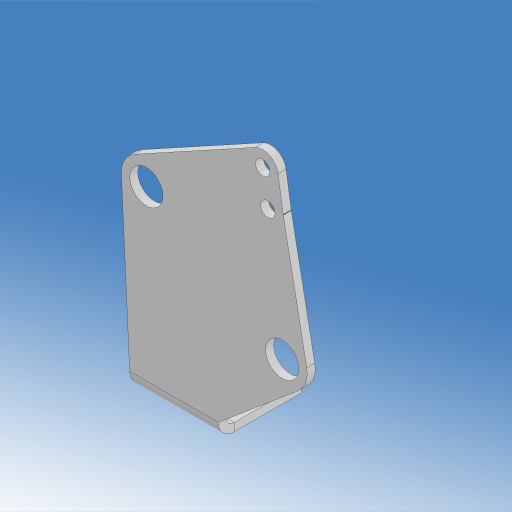
# Autodesk Inventor part: GearsMount
Saved by Autodesk Inventor 2024 (Build 280153000, 153)
## iProperties
Created: 2024-03-12
Part Number: GearsMount
Material: Generic
Document SubType Name: Sheet Metal
Designer: seene
Density: 1 g/cm^3
Sheet Metal Rule: Default
Appearance: Default
Author: seene
Autodesk Inventor part; units mm, degrees
ref_plane "YZ Plane" through (0, 0, 0) normal (1, 0, 0) x (0, 1, 0)
ref_plane "XZ Plane" through (0, 0, 0) normal (0, 1, 0) x (-1, 0, 0)
ref_plane "XY Plane" through (0, 0, 0) normal (0, 0, 1) x (1, 0, 0)
sketch "Sketch1" plane through (0, 0, 0) normal (0, 0, 1) x (1, 0, 0)
  circle A0 centre (6.35, 64.0658) radius 6.35
  circle A1 centre (58.0536, 32.9878) radius 6.35
  line L0 (0, 0) -> (33.7266, 0)
  circle A2 centre (50.6167, 92.4839) radius 2.7589
  circle A3 centre (52.5819, 79.7839) radius 2.7589
  line L1 (0, 0) -> (0, 86.6758) construction
  dimension "d12" = 12.7
  dimension "d13" = 12.7
  dimension "d15" = 51.7036
  dimension "d16" = 31.078
  dimension "d18" = 32.9877
  dimension "d19" = 24.327
  dimension "d20" = 5.5178
  dimension "d21" = 5.5178
  dimension "d22" = 46.7962
  dimension "d23" = 5.4717
  dimension "d24" = 1.9652
  dimension "d25" = 12.7
  constraints: 4 centre point, 4 end point, 1 horizontal, 1 tangent, 1 vertical
  measures "d12" diameter of A0
  measures "d13" diameter of A1
  measures "d15" horizontal distance of A1.centre A0.centre
  measures "d16" vertical distance of A1.centre A0.centre
  measures "d18" distance from line of L0 A1.centre
  measures "d19" horizontal distance of A1.centre L0.end
  measures "d20" diameter of A2
  measures "d21" diameter of A3
  measures "d22" vertical distance of A1.centre A3.centre
  measures "d23" horizontal distance of A1.centre A3.centre
  measures "d24" horizontal distance of A3.centre A2.centre
  measures "d25" vertical distance of A3.centre A2.centre
sketch "Sketch3" plane through (0, 0, 0) normal (0, 0, 1) x (1, 0, 0)
  circle A0 centre (6.35, 64.0658) radius 6.35
  circle A1 centre (50.6167, 92.4839) radius 2.7589
  circle A2 centre (52.5819, 79.7839) radius 2.7589
  circle A3 centre (58.0536, 32.9878) radius 6.35
  circle A4 centre (6.35, 64.0658) radius 9.525
  circle A5 centre (58.0536, 32.9878) radius 9.525
  circle A6 centre (52.5819, 79.7839) radius 5.9339
  circle A7 centre (50.6167, 92.4839) radius 5.9339
  line L0 (0, 0) -> (-3.1632, 63.5926)
  line L1 (33.7266, 0) -> (64.1959, 25.7078)
  line L2 (1.7635, 72.4138) -> (47.7594, 97.6846)
  line L3 (56.4808, 93.3913) -> (58.446, 80.6913)
  line L4 (58.406, 80.9203) -> (67.4023, 34.8118)
  line L5 (6.35, 64.0658) -> (58.0536, 32.9878) construction
  line L6 (58.0536, 32.9878) -> (52.5819, 79.7839) construction
  line L7 (52.5819, 79.7839) -> (50.6167, 92.4839) construction
  line L8 (50.6167, 92.4839) -> (6.35, 64.0658) construction
  line L9 (52.5819, 79.7839) -> (6.35, 64.0658) construction
  line L10 (0, 0) -> (33.7266, 0)
  line L11 (0, 0) -> (33.7266, 0)
  line L12 (33.7266, 0) -> (33.7266, -31.75)
  line L13 (33.7266, -31.75) -> (0, -31.75)
  line L14 (0, -31.75) -> (0, 0)
  point P0 (58.4282, 80.8062)
  dimension "d27" = 3.175
  dimension "d28" = 3.175
  dimension "d29" = 3.175
  dimension "d30" = 3.175
  dimension "d33" = 31.75
  measures "d27" radial gap between concentric circles of A0 A4
  measures "d28" radial gap between concentric circles of A3 A5
  measures "d29" radial gap between concentric circles of A7 A1
  measures "d30" radial gap between concentric circles of A6 A2
  measures "d33" distance of L13.end L10.start
extrude "Plate3" add sketch "Sketch3" along normal blind 3.048 contours A4 | A6 | A4 L2 A7 L3 L4 A5 L1 L10 L0 | A7 | A5
sketch "Sketch4" plane through (0, -3.048, -3.048) normal (0, -1, 0) x (1, 0, 0)
  line L0 (33.7266, 0) -> (0, 0)
  line L1 (0, 0) -> (0, -25.654)
  line L2 (0, -25.654) -> (33.7266, -25.654)
  line L3 (33.7266, -25.654) -> (33.7266, 0)
  constraints: 6 end point, 1 horizontal, 1 perpendicular, 1 vertical
edge flange "Flange1" height 31.75 angle 90 thickness 3.048 bend radius 3.048 thickness toward (0, -1, 0) relief tear relief width 3.048 relief depth 1.524 edges at (16.8633, 0, 0) wall of the first edge with corners at (33.7266, -3.048, -3.048) (0, -3.048, -3.048) (0, -3.048, -28.702) (33.7266, -3.048, -28.702)
bend "Bend3"
corner "Corner1"
equation "\"d21\" = d20"
equation "\"d28\" = d27"
equation "\"d29\" = d27"
equation "\"d30\" = d27"
equation "\"d31\" = Thickness"
equation "\"d34\" = BendReliefWidth"
equation "\"d35\" = BendReliefDepth"
equation "\"d36\" = MinimumRemnant"
equation "\"d37\" = TransitionRadius"
equation "\"d40\" = BendRadius"
equation "\"d41\" = CornerReliefSize"
equation "\"d42\" = GapSize"
equation "\"d43\" = JacobiRadiusSize"
equation "\"BendRadius\" = Thickness"
equation "\"BendReliefWidth\" = Thickness"
equation "\"BendReliefDepth\" = 0.5 * Thickness"
equation "\"CornerReliefSize\" = 4 * Thickness"
equation "\"MinimumRemnant\" = 2 * Thickness"
equation "\"TransitionRadius\" = BendRadius"
equation "\"JacobiRadiusSize\" = BendRadius"
equation "\"GapSize\" = Thickness"
equation "\"Thickness\" = 3.048"
body "Solid2"
